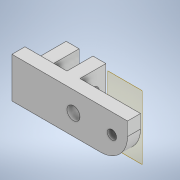
# Autodesk Inventor part: adapter_1
Saved by Autodesk Inventor 2020.1 (Build 241239000, 239)
## iProperties
Created: 2019-10-23
Part Number: adapter_1
Material: Generic
Document SubType Name: Modeling
Designer: jesse
Density: 1 g/cm^3
Appearance: Default
Author: jesse
## iProperties of the stored document _3DPrint.ipt
Created: 2019-10-25
Part Number: _3DPrint
Material: Generic
Document SubType Name: Modeling
Designer: jesse
Density: 1 g/cm^3
Appearance: Default
Author: jesse
Autodesk Inventor part; units mm, degrees
ref_plane "YZ Plane" through (0, 0, 0) normal (1, 0, 0) x (0, 1, 0)
ref_plane "XZ Plane" through (0, 0, 0) normal (0, 1, 0) x (-1, 0, 0)
ref_plane "XY Plane" through (0, 0, 0) normal (0, 0, 1) x (1, 0, 0)
ref_plane "Work Plane1" through (0, 0, 0) normal (0, 0, 1) x (1, 0, 0)
sketch "Sketch1" plane through (0, 0, 0) normal (0, 0, 1) x (1, 0, 0)
  line L0 (31.75, -13.716) -> (31.75, -6.096) projected
  arc A0 (25.146, -20.32) -> (31.75, -13.716) centre (25.146, -13.716) ccw projected
  line L1 (24.13, -20.32) -> (25.146, -20.32) projected
  circle A1 centre (27.94, -15.24) radius 1.1303 projected
  line L2 (31.75, -6.096) -> (31.75, -10.4198)
  line L3 (31.75, -10.4198) -> (24.13, -10.4198)
  line L4 (24.13, -10.4198) -> (24.13, -20.32)
  point P0 (0, 0)
  constraints: 6 end point, 1 perpendicular, 1 point on line, 1 vertical
extrude "Extrusion1" add sketch "Sketch1" along normal blind 3.175
move faces "Move1" translate (-20.6502, 0, 0) faces at (24.13, -13.7199, 1.0583)
sketch "Sketch2" plane through (0, 0, 0) normal (0, 0, -1) x (-1, 0, 0)
  line L0 (-13.6627, -7.7169) -> (-13.6627, -20.1208) projected
  line L1 (-10.4877, -7.7169) -> (-10.4877, -20.1208) projected
  line L2 (-3.4798, -20.32) -> (-25.146, -20.32) projected
  line L3 (-10.3877, -20.32) -> (-7.2127, -20.32)
  line L4 (-7.2127, -20.32) -> (-7.2127, -10.5651)
  line L5 (-7.2127, -10.5651) -> (-10.3877, -10.5651)
  line L6 (-10.3877, -10.5651) -> (-10.3877, -20.32)
  line L7 (-31.75, -10.4198) -> (-3.4798, -10.4198) projected
  line L8 (-13.7627, -20.32) -> (-16.9377, -20.32)
  line L9 (-16.9377, -20.32) -> (-16.9377, -10.4198)
  line L10 (-16.9377, -10.4198) -> (-13.7627, -10.4198)
  line L11 (-13.7627, -10.4198) -> (-13.7627, -20.32)
  point P0 (0, 0)
  dimension "d5" = 0.1
  dimension "d6" = 0.1
  dimension "d7" = 3.175
  dimension "d8" = 3.175
  constraints: 16 end point, 4 parallel, 3 point on line, 2 horizontal, 2 perpendicular
  measures "d5" distance between parallel lines of L6 L1
  measures "d6" distance between parallel lines of L11 L0
  measures "d7" distance between parallel lines of L11 L9
  measures "d8" distance between parallel lines of L6 L4
extrude "Extrusion2" add sketch "Sketch2" along normal blind 6.35
sketch "Sketch3" plane through (6.6139, -20.32, 0) normal (-1, 0, 0) x (0, 0, 1)
  line L0 (0, 9.7549) -> (0, 0) construction
  line L1 (0, 9.7549) -> (-6.35, 9.7549) construction
  line L2 (-6.35, 0) -> (-6.35, 9.7549) construction
  line L3 (0, 0) -> (-6.35, 0) construction
  line L4 (0, 0) -> (-6.35, 9.7549) construction
  circle A0 centre (-3.175, 4.8775) radius 1.5875
  point P0 (0, 20.32)
  dimension "d11" = 3.175
  constraints: 2 end point, 1 centre point, 1 midpoint
  measures "d11" diameter of A0
extrude "Extrusion3" [suppressed]
sketch "Sketch4" plane through (0, 0, 0) normal (0, 0, -1) x (-1, 0, 0)
  line L0 (-16.9377, -20.32) -> (-16.9377, -10.4198) construction
  line L1 (-16.9377, -15.3699) -> (-22.7751, -15.3699) construction
  circle A0 centre (-18.5252, -15.3699) radius 1.5875
  point P0 (0, 0)
  dimension "d17" = 3.175
  constraints: 2 end point, 1 centre point, 1 horizontal, 1 midpoint, 1 point on line, 1 tangent
  measures "d17" diameter of A0
extrude "Extrusion4" cut sketch "Sketch4" against normal blind 12.7
sketch "Sketch5" plane through (7.2127, -20.32, 0) normal (-1, 0, 0) x (0, 0, 1)
  line L0 (0, 9.7549) -> (0, 0) projected
  line L1 (-6.35, 0) -> (-6.35, 9.7549) projected
  line L2 (0, 9.7549) -> (-6.35, 0) construction
  circle A0 centre (-3.175, 4.8775) radius 1.5875
  point P0 (0, 20.32)
  dimension "d20" = 3.175
  constraints: 2 end point, 1 centre point, 1 midpoint
  measures "d20" diameter of A0
extrude "Extrusion5" cut sketch "Sketch5" against normal blind 17.4625
body "Solid1"
